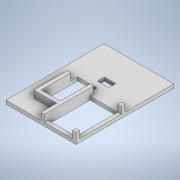
# Autodesk Inventor part: chassis_top
Saved by Autodesk Inventor 2022 (Build 260153000, 153)
## iProperties
Created: 2021-04-16
Part Number: chassis_top
Material: Generic
Document SubType Name: Modeling
Designer: kevin
Density: 1 g/cm^3
Appearance: Default
Author: kevin
Autodesk Inventor part; units mm, degrees
ref_plane "YZ Plane" through (0, 0, 0) normal (1, 0, 0) x (0, 1, 0)
ref_plane "XZ Plane" through (0, 0, 0) normal (0, 1, 0) x (-1, 0, 0)
ref_plane "XY Plane" through (0, 0, 0) normal (0, 0, 1) x (1, 0, 0)
sketch "Sketch1" plane through (0, 0, 0) normal (0, 1, 0) x (-1, 0, 0)
  line L0 (63.5, 88.9) -> (-63.5, 88.9)
  line L1 (-63.5, 88.9) -> (-63.5, -88.9)
  line L2 (-63.5, -88.9) -> (63.5, -88.9)
  line L3 (63.5, -88.9) -> (63.5, 88.9)
  line L4 (63.5, 88.9) -> (-63.5, -88.9) construction
  line L5 (-63.5, 88.9) -> (63.5, -88.9) construction
  point P0 (0, 0)
  dimension "d0" = 177.8
  dimension "d1" = 127
  constraints: 12 end point, 2 midpoint, 2 parallel, 1 horizontal, 1 perpendicular
  measures "d0" distance of L2.end L0.start
  measures "d1" distance of L0.start L0.end
extrude "main plate" add sketch "Sketch1" along normal blind 6.35
sketch "Sketch4" plane through (0, 6.35, 0) normal (0, 1, 0) x (1, 0, 0)
  line L0 (63.5, -88.9) -> (63.5, 88.9) projected
  line L1 (63.5, -88.9) -> (57.15, -88.9)
  line L2 (57.15, -88.9) -> (57.15, -82.55)
  line L3 (57.15, -82.55) -> (63.5, -82.55)
  line L4 (63.5, -82.55) -> (63.5, -88.9)
  line L5 (57.15, -82.55) -> (6.35, -82.55) construction
  line L6 (57.15, -82.55) -> (57.15, -6.35) construction
  line L7 (57.15, -6.35) -> (63.5, -6.35)
  line L8 (63.5, -6.35) -> (63.5, 0)
  line L9 (63.5, 0) -> (57.15, 0)
  line L10 (57.15, 0) -> (57.15, -6.35)
  line L11 (-63.5, -88.9) -> (63.5, -88.9) projected
  line L12 (6.35, -82.55) -> (0, -82.55)
  line L13 (0, -82.55) -> (0, -88.9)
  line L14 (0, -88.9) -> (6.35, -88.9)
  line L15 (6.35, -88.9) -> (6.35, -82.55)
  line L16 (0, 0) -> (6.35, 0)
  line L17 (6.35, 0) -> (6.35, -6.35)
  line L18 (6.35, -6.35) -> (0, -6.35)
  line L19 (0, -6.35) -> (0, 0)
  line L20 (6.35, -6.35) -> (0, -6.35)
  line L21 (0, -6.35) -> (0, -82.55)
  line L22 (0, -82.55) -> (6.35, -82.55)
  line L23 (6.35, -82.55) -> (6.35, -6.35)
  dimension "d12" = 6.35
  dimension "d13" = 6.35
  dimension "d14" = 50.8
  dimension "d15" = 76.2
  constraints: 44 end point, 10 parallel, 6 horizontal, 5 perpendicular, 2 midpoint, 2 point on line, 1 vertical
  measures "d12" distance of L0.start L1.end
  measures "d13" distance of L1.end L2.end
  measures "d14" distance of L2.end L5.end
  measures "d15" distance of L2.end L6.end
extrude "battery standoffs" add sketch "Sketch4" along normal blind 12.7
sketch "Sketch5" plane through (0, 6.35, 0) normal (0, 1, 0) x (1, 0, 0)
  line L0 (-34.925, -6.35) -> (0, -6.35)
  line L1 (0, -6.35) -> (0, -53.975)
  line L2 (0, -53.975) -> (-34.925, -53.975)
  line L3 (-34.925, -53.975) -> (-34.925, -6.35)
  line L4 (-34.925, -6.35) -> (0, -6.35)
  line L5 (0, -6.35) -> (0, -53.975)
  line L6 (0, -53.975) -> (-34.925, -53.975)
  line L7 (-34.925, -53.975) -> (-34.925, -6.35)
  point P0 (0, 0)
  dimension "d18" = 34.925
  dimension "d19" = 47.625
  constraints: 16 end point, 4 parallel, 2 horizontal, 2 perpendicular
  measures "d18" distance of L1.end L2.end
  measures "d19" distance of L2.end L0.start
extrude "breadboard hole" cut sketch "Sketch5" against normal blind 6.35
sketch "Sketch6" plane through (0, 6.35, 0) normal (0, 1, 0) x (1, 0, 0)
  line L0 (6.35, 0) -> (6.35, -6.35) projected
  line L1 (6.35, -6.35) -> (57.15, -6.35)
  line L2 (57.15, -6.35) -> (57.15, -82.55)
  line L3 (57.15, -82.55) -> (6.35, -82.55)
  line L4 (6.35, -82.55) -> (6.35, -6.35)
  point P0 (0, 0)
  constraints: 8 end point, 2 parallel, 1 horizontal, 1 perpendicular
extrude "battery hole" cut sketch "Sketch6" against normal blind 6.35
sketch "Sketch9" plane through (0, 6.35, 0) normal (0, 1, 0) x (1, 0, 0)
  line L0 (0, -53.975) -> (0, -6.35) projected
  line L1 (0, -53.975) -> (-34.925, -53.975)
  line L2 (-34.925, -53.975) -> (-34.925, -60.325)
  line L3 (-34.925, -60.325) -> (0, -60.325)
  line L4 (0, -60.325) -> (0, -53.975)
  line L5 (-34.925, -60.325) -> (-41.275, -60.325)
  line L6 (-41.275, -60.325) -> (-41.275, 0)
  line L7 (-41.275, 0) -> (-34.925, 0)
  line L8 (-34.925, 0) -> (-34.925, -60.325)
  line L9 (0, 0) -> (0, -6.35)
  line L10 (-34.925, -6.35) -> (-34.925, 0)
  point P0 (0, 0)
  constraints: 20 end point, 5 parallel, 2 horizontal, 2 perpendicular, 1 point on line
extrude "breadboard standoffs" add sketch "Sketch9" along normal blind 12.7
sketch "Sketch10" plane through (0, 6.35, 0) normal (0, 1, 0) x (1, 0, 0)
  line L0 (-34.925, 0) -> (-34.925, -6.35) projected
  line L1 (-34.925, -6.35) -> (0, -6.35)
  line L2 (0, -6.35) -> (0, 12.7)
  line L3 (0, 12.7) -> (-34.925, 12.7)
  line L4 (-34.925, 12.7) -> (-34.925, -6.35)
  point P0 (0, 0)
  constraints: 8 end point, 2 parallel, 1 horizontal, 1 perpendicular
extrude "wiring hole" cut sketch "Sketch10" against normal blind 6.35
sketch "Sketch11" plane through (0, 6.35, 0) normal (0, 1, 0) x (1, 0, 0)
  line L0 (-10.3188, 36.5125) -> (10.3187, 36.5125)
  line L1 (10.3187, 36.5125) -> (10.3187, 23.8125)
  line L2 (10.3187, 23.8125) -> (-10.3187, 23.8125)
  line L3 (-10.3187, 23.8125) -> (-10.3188, 36.5125)
  line L4 (-10.3188, 36.5125) -> (10.3187, 23.8125) construction
  line L5 (10.3187, 36.5125) -> (-10.3187, 23.8125) construction
  point P0 (0, 0)
  point P1 (0, 30.1625)
  dimension "d28" = 12.7
  dimension "d29" = 20.6375
  constraints: 12 end point, 2 midpoint, 2 parallel, 1 horizontal, 1 perpendicular
  measures "d28" distance of L0.end L1.end
  measures "d29" distance of L0.start L0.end
extrude "power switch mount" cut sketch "Sketch11" against normal blind 6.35
body "Solid1"
